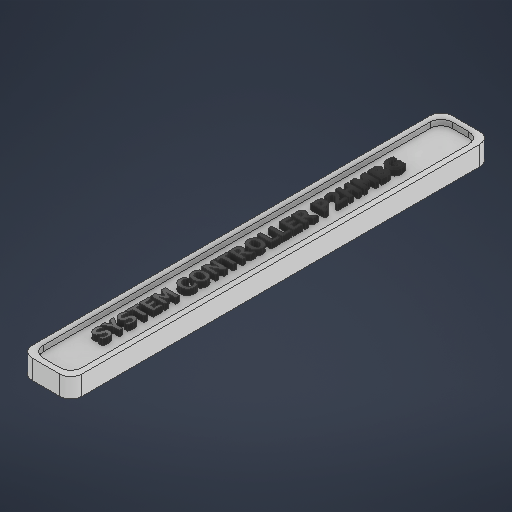
# Autodesk Inventor part: ELEMENT P2HMBG
Saved by Autodesk Inventor 2026.3 (Build 303398000, 398)
## iProperties
Created: 2026-06-09
Part Number: ELEMENT P2HMBG
Material: Generic
Document SubType Name: Modeling
Designer: ilyas
Density: 1 g/cm^3
Appearance: Default
Author: ilyas
Autodesk Inventor part; units mm, degrees
ref_plane "YZ Plane" through (0, 0, 0) normal (1, 0, 0) x (0, 1, 0)
ref_plane "XZ Plane" through (0, 0, 0) normal (0, 1, 0) x (-1, 0, 0)
ref_plane "XY Plane" through (0, 0, 0) normal (0, 0, 1) x (1, 0, 0)
sketch "Sketch1" plane through (0, 0, 0) normal (0, 1, 0) x (-1, 0, 0)
  line L0 (-4.5, 38) -> (4.5, 38)
  line L1 (4.5, 38) -> (4.5, -38)
  line L2 (4.5, -38) -> (-4.5, -38)
  line L3 (-4.5, -38) -> (-4.5, 38)
  line L4 (-4.5, 38) -> (4.5, -38) construction
  line L5 (4.5, 38) -> (-4.5, -38) construction
  point P0 (0, 0)
  dimension "d0" = 9
  dimension "d1" = 76
  constraints: 12 end point, 2 midpoint, 2 parallel, 1 horizontal, 1 perpendicular
  measures "d0" distance of L1.end L2.end
  measures "d1" distance of L0.end L1.end
extrude "Extrusion1" add sketch "Sketch1" along normal blind 2.5
sketch "Sketch2" plane through (0, 2.5, 0) normal (0, 1, 0) x (1, 0, 0)
  line L0 (4.5, -38) -> (-4.5, -38)
  line L1 (-4.5, -38) -> (-4.5, 38)
  line L2 (-4.5, 38) -> (4.5, 38)
  line L3 (4.5, 38) -> (4.5, -38)
  line L4 (4.5, -38) -> (-4.5, 38) construction
  line L5 (-4.5, -38) -> (4.5, 38) construction
  line L6 (-3.5, 37) -> (-3.5, -37)
  line L7 (-3.5, -37) -> (3.5, -37)
  line L8 (3.5, -37) -> (3.5, 37)
  line L9 (3.5, 37) -> (-3.5, 37)
  point P0 (0, 0)
  dimension "d4" = 9
  dimension "d5" = 76
  dimension "d6" = 1
  constraints: 20 end point, 4 parallel, 2 midpoint, 2 perpendicular, 1 horizontal, 3 other
  measures "d4" distance of L1.end L2.end
  measures "d5" distance of L0.end L1.end
  measures "d6" distance between parallel lines of L1 L6
emboss "Emboss1" sketch "Sketch2" operation add depth 1 direction (0, -1, 0)
sketch "Sketch3" plane through (0, 2.5, 0) normal (0, 1, 0) x (1, 0, 0)
  line L0 (-7.0021, -29.5186) -> (-7.0021, 27.1388) construction
  line L1 (-7.0021, 27.1388) -> (6.5444, 27.1388) construction
  line L2 (6.5444, 27.1388) -> (6.5444, -29.5186) construction
  line L3 (6.5444, -29.5186) -> (-7.0021, -29.5186) construction
  spline S0 degree 2 poles (1.0865, -27.7879) (1.0865, -28.0801) (0.9732, -28.5206) (0.8909, -28.71) knots 0 0 0 1 2 2 2
  line L4 (0.8909, -28.71) -> (0.2858, -28.71)
  line L5 (0.2858, -28.71) -> (0.2858, -28.6524)
  spline S1 degree 2 poles (0.2858, -28.6524) (0.4484, -28.4609) (0.6233, -28.0019) (0.6233, -27.7858) knots 0 0 0 1 2 2 2
  spline S2 degree 2 poles (0.6233, -27.7858) (0.6233, -27.7302) (0.5986, -27.5511) (0.5739, -27.4976) knots 0 0 0 1 2 2 2
  spline S3 degree 2 poles (0.5739, -27.4976) (0.5451, -27.4318) (0.4401, -27.3391) (0.3557, -27.3391) knots 0 0 0 1 2 2 2
  spline S4 degree 2 poles (0.3557, -27.3391) (0.259, -27.3391) (0.1396, -27.4894) (0.1129, -27.5923) knots 0 0 0 1 2 2 2
  spline S5 degree 2 poles (0.1129, -27.5923) (0.0779, -27.722) (0.0182, -28.0163) (-0.0271, -28.146) knots 0 0 0 1 2 2 2
  spline S6 degree 2 poles (-0.0271, -28.146) (-0.13, -28.4404) (-0.482, -28.6956) (-0.7455, -28.6956) knots 0 0 0 1 2 2 2
  spline S7 degree 2 poles (-0.7455, -28.6956) (-1.1016, -28.6956) (-1.5441, -28.0925) (-1.5441, -27.6397) knots 0 0 0 1 2 2 2
  spline S8 degree 2 poles (-1.5441, -27.6397) (-1.5441, -27.4132) (-1.4515, -26.9645) (-1.3733, -26.7875) knots 0 0 0 1 2 2 2
  line L6 (-1.3733, -26.7875) -> (-0.7928, -26.7875)
  line L7 (-0.7928, -26.7875) -> (-0.7928, -26.8431)
  spline S9 degree 2 poles (-0.7928, -26.8431) (-0.9143, -26.9851) (-1.081, -27.3927) (-1.081, -27.6067) knots 0 0 0 1 2 2 2
  spline S10 degree 2 poles (-1.081, -27.6067) (-1.081, -27.6911) (-1.0563, -27.8228) (-1.0233, -27.8969) knots 0 0 0 1 2 2 2
  spline S11 degree 2 poles (-1.0233, -27.8969) (-0.9966, -27.9566) (-0.8896, -28.0431) (-0.8237, -28.0431) knots 0 0 0 1 2 2 2
  spline S12 degree 2 poles (-0.8237, -28.0431) (-0.7249, -28.0431) (-0.6117, -27.9052) (-0.5664, -27.7076) knots 0 0 0 1 2 2 2
  spline S13 degree 2 poles (-0.5664, -27.7076) (-0.5376, -27.58) (-0.482, -27.3433) (-0.4347, -27.2074) knots 0 0 0 1 2 2 2
  spline S14 degree 2 poles (-0.4347, -27.2074) (-0.3379, -26.9439) (-0.0168, -26.6866) (0.2467, -26.6866) knots 0 0 0 1 2 2 2
  spline S15 degree 2 poles (0.2467, -26.6866) (0.6254, -26.6866) (1.0865, -27.2815) (1.0865, -27.7879) knots 0 0 0 1 2 2 2
  line L8 (-1.4988, -24.2475) -> (-0.0189, -25.1244)
  line L9 (-0.0189, -25.1244) -> (1.0412, -25.1244)
  line L10 (1.0412, -25.1244) -> (1.0412, -25.7624)
  line L11 (1.0412, -25.7624) -> (0.012, -25.7624)
  line L12 (0.012, -25.7624) -> (-1.4988, -26.6537)
  line L13 (-1.4988, -26.6537) -> (-1.4988, -25.9271)
  line L14 (-1.4988, -25.9271) -> (-0.5932, -25.431)
  line L15 (-0.5932, -25.431) -> (-1.4988, -24.9515)
  line L16 (-1.4988, -24.9515) -> (-1.4988, -24.2475)
  spline S16 degree 2 poles (1.0865, -23.2327) (1.0865, -23.525) (0.9732, -23.9655) (0.8909, -24.1549) knots 0 0 0 1 2 2 2
  line L17 (0.8909, -24.1549) -> (0.2858, -24.1549)
  line L18 (0.2858, -24.1549) -> (0.2858, -24.0972)
  spline S17 degree 2 poles (0.2858, -24.0972) (0.4484, -23.9058) (0.6233, -23.4468) (0.6233, -23.2307) knots 0 0 0 1 2 2 2
  spline S18 degree 2 poles (0.6233, -23.2307) (0.6233, -23.1751) (0.5986, -22.996) (0.5739, -22.9425) knots 0 0 0 1 2 2 2
  spline S19 degree 2 poles (0.5739, -22.9425) (0.5451, -22.8766) (0.4401, -22.784) (0.3557, -22.784) knots 0 0 0 1 2 2 2
  spline S20 degree 2 poles (0.3557, -22.784) (0.259, -22.784) (0.1396, -22.9343) (0.1129, -23.0372) knots 0 0 0 1 2 2 2
  spline S21 degree 2 poles (0.1129, -23.0372) (0.0779, -23.1669) (0.0182, -23.4612) (-0.0271, -23.5909) knots 0 0 0 1 2 2 2
  spline S22 degree 2 poles (-0.0271, -23.5909) (-0.13, -23.8852) (-0.482, -24.1405) (-0.7455, -24.1405) knots 0 0 0 1 2 2 2
  spline S23 degree 2 poles (-0.7455, -24.1405) (-1.1016, -24.1405) (-1.5441, -23.5374) (-1.5441, -23.0845) knots 0 0 0 1 2 2 2
  spline S24 degree 2 poles (-1.5441, -23.0845) (-1.5441, -22.8581) (-1.4515, -22.4094) (-1.3733, -22.2324) knots 0 0 0 1 2 2 2
  line L19 (-1.3733, -22.2324) -> (-0.7928, -22.2324)
  line L20 (-0.7928, -22.2324) -> (-0.7928, -22.288)
  spline S25 degree 2 poles (-0.7928, -22.288) (-0.9143, -22.43) (-1.081, -22.8375) (-1.081, -23.0516) knots 0 0 0 1 2 2 2
  spline S26 degree 2 poles (-1.081, -23.0516) (-1.081, -23.136) (-1.0563, -23.2677) (-1.0233, -23.3418) knots 0 0 0 1 2 2 2
  spline S27 degree 2 poles (-1.0233, -23.3418) (-0.9966, -23.4015) (-0.8896, -23.488) (-0.8237, -23.488) knots 0 0 0 1 2 2 2
  spline S28 degree 2 poles (-0.8237, -23.488) (-0.7249, -23.488) (-0.6117, -23.3501) (-0.5664, -23.1525) knots 0 0 0 1 2 2 2
  spline S29 degree 2 poles (-0.5664, -23.1525) (-0.5376, -23.0248) (-0.482, -22.7881) (-0.4347, -22.6523) knots 0 0 0 1 2 2 2
  spline S30 degree 2 poles (-0.4347, -22.6523) (-0.3379, -22.3888) (-0.0168, -22.1315) (0.2467, -22.1315) knots 0 0 0 1 2 2 2
  spline S31 degree 2 poles (0.2467, -22.1315) (0.6254, -22.1315) (1.0865, -22.7264) (1.0865, -23.2327) knots 0 0 0 1 2 2 2
  line L21 (1.0412, -21.3164) -> (-1.0151, -21.3164)
  line L22 (-1.0151, -21.3164) -> (-1.0151, -22.0677)
  line L23 (-1.0151, -22.0677) -> (-1.4988, -22.0677)
  line L24 (-1.4988, -22.0677) -> (-1.4988, -19.927)
  line L25 (-1.4988, -19.927) -> (-1.0151, -19.927)
  line L26 (-1.0151, -19.927) -> (-1.0151, -20.6783)
  line L27 (-1.0151, -20.6783) -> (1.0412, -20.6783)
  line L28 (1.0412, -20.6783) -> (1.0412, -21.3164)
  line L29 (1.0412, -19.6656) -> (-1.4988, -19.6656)
  line L30 (-1.4988, -19.6656) -> (-1.4988, -17.949)
  line L31 (-1.4988, -17.949) -> (-1.0151, -17.949)
  line L32 (-1.0151, -17.949) -> (-1.0151, -19.0316)
  line L33 (-1.0151, -19.0316) -> (-0.5685, -19.0316)
  line L34 (-0.5685, -19.0316) -> (-0.5685, -18.0333)
  line L35 (-0.5685, -18.0333) -> (-0.0847, -18.0333)
  line L36 (-0.0847, -18.0333) -> (-0.0847, -19.0316)
  line L37 (-0.0847, -19.0316) -> (0.5575, -19.0316)
  line L38 (0.5575, -19.0316) -> (0.5575, -17.949)
  line L39 (0.5575, -17.949) -> (1.0412, -17.949)
  line L40 (1.0412, -17.949) -> (1.0412, -19.6656)
  line L41 (1.0412, -14.9232) -> (1.0412, -15.5572)
  line L42 (1.0412, -15.5572) -> (-0.6426, -15.5572)
  line L43 (-0.6426, -15.5572) -> (0.4443, -16.0182)
  line L44 (0.4443, -16.0182) -> (0.4443, -16.4546)
  line L45 (0.4443, -16.4546) -> (-0.6426, -16.9157)
  line L46 (-0.6426, -16.9157) -> (1.0412, -16.9157)
  line L47 (1.0412, -16.9157) -> (1.0412, -17.5167)
  line L48 (1.0412, -17.5167) -> (-1.4988, -17.5167)
  line L49 (-1.4988, -17.5167) -> (-1.4988, -16.7819)
  line L50 (-1.4988, -16.7819) -> (-0.2453, -16.2179)
  line L51 (-0.2453, -16.2179) -> (-1.4988, -15.658)
  line L52 (-1.4988, -15.658) -> (-1.4988, -14.9232)
  line L53 (-1.4988, -14.9232) -> (1.0412, -14.9232)
  spline S32 degree 2 poles (1.0906, -12.2782) (1.0906, -12.8504) (0.399, -13.5215) (-0.2268, -13.5215) knots 0 0 0 1 2 2 2
  spline S33 degree 2 poles (-0.2268, -13.5215) (-0.8299, -13.5215) (-1.5482, -12.8484) (-1.5482, -12.2762) knots 0 0 0 1 2 2 2
  spline S34 degree 2 poles (-1.5482, -12.2762) (-1.5482, -12.1259) (-1.5132, -11.883) (-1.4844, -11.7719) knots 0 0 0 1 2 2 2
  spline S35 degree 2 poles (-1.4844, -11.7719) (-1.4577, -11.6854) (-1.3692, -11.4816) (-1.3362, -11.4178) knots 0 0 0 1 2 2 2
  line L54 (-1.3362, -11.4178) -> (-0.7311, -11.4178)
  line L55 (-0.7311, -11.4178) -> (-0.7311, -11.4816)
  spline S36 degree 2 poles (-0.7311, -11.4816) (-0.7722, -11.529) (-0.8875, -11.6689) (-0.941, -11.7575) knots 0 0 0 1 2 2 2
  spline S37 degree 2 poles (-0.941, -11.7575) (-0.9966, -11.846) (-1.0727, -12.058) (-1.0727, -12.1753) knots 0 0 0 1 2 2 2
  spline S38 degree 2 poles (-1.0727, -12.1753) (-1.0727, -12.3132) (-0.9863, -12.5417) (-0.8772, -12.6467) knots 0 0 0 1 2 2 2
  spline S39 degree 2 poles (-0.8772, -12.6467) (-0.7805, -12.7413) (-0.4491, -12.8628) (-0.2247, -12.8628) knots 0 0 0 1 2 2 2
  spline S40 degree 2 poles (-0.2247, -12.8628) (0.012, -12.8628) (0.3352, -12.7372) (0.434, -12.6343) knots 0 0 0 1 2 2 2
  spline S41 degree 2 poles (0.434, -12.6343) (0.5307, -12.5355) (0.6151, -12.2926) (0.6151, -12.1712) knots 0 0 0 1 2 2 2
  spline S42 degree 2 poles (0.6151, -12.1712) (0.6151, -12.0456) (0.5307, -11.8171) (0.4792, -11.7389) knots 0 0 0 1 2 2 2
  spline S43 degree 2 poles (0.4792, -11.7389) (0.4278, -11.6525) (0.3187, -11.5228) (0.2755, -11.4755) knots 0 0 0 1 2 2 2
  line L56 (0.2755, -11.4755) -> (0.2755, -11.4178)
  line L57 (0.2755, -11.4178) -> (0.8724, -11.4178)
  spline S44 degree 2 poles (0.8724, -11.4178) (0.9053, -11.4878) (0.9877, -11.671) (1.0165, -11.7698) knots 0 0 0 1 2 2 2
  spline S45 degree 2 poles (1.0165, -11.7698) (1.0535, -11.8892) (1.0906, -12.0971) (1.0906, -12.2782) knots 0 0 0 1 2 2 2
  spline S46 degree 2 poles (-0.2288, -8.7296) (0.3887, -8.7296) (1.0947, -9.3883) (1.0947, -9.9605) knots 0 0 0 1 2 2 2
  spline S47 degree 2 poles (1.0947, -9.9605) (1.0947, -10.5348) (0.3804, -11.1893) (-0.2288, -11.1893) knots 0 0 0 1 2 2 2
  spline S48 degree 2 poles (-0.2288, -11.1893) (-0.8402, -11.1893) (-1.5523, -10.5348) (-1.5523, -9.9605) knots 0 0 0 1 2 2 2
  spline S49 degree 2 poles (-1.5523, -9.9605) (-1.5523, -9.3883) (-0.8443, -8.7296) (-0.2288, -8.7296) knots 0 0 0 1 2 2 2
  spline S50 degree 2 poles (-0.2288, -9.3883) (-0.4573, -9.3883) (-0.7763, -9.4809) (-0.8772, -9.5612) knots 0 0 0 1 2 2 2
  spline S51 degree 2 poles (-0.8772, -9.5612) (-0.9822, -9.6415) (-1.0727, -9.8473) (-1.0727, -9.9585) knots 0 0 0 1 2 2 2
  spline S52 degree 2 poles (-1.0727, -9.9585) (-1.0727, -10.0758) (-0.9884, -10.2672) (-0.8813, -10.3557) knots 0 0 0 1 2 2 2
  spline S53 degree 2 poles (-0.8813, -10.3557) (-0.7825, -10.4339) (-0.4552, -10.5307) (-0.2288, -10.5307) knots 0 0 0 1 2 2 2
  spline S54 degree 2 poles (-0.2288, -10.5307) (0.0058, -10.5307) (0.3146, -10.438) (0.4196, -10.3578) knots 0 0 0 1 2 2 2
  spline S55 degree 2 poles (0.4196, -10.3578) (0.5245, -10.2775) (0.6151, -10.0696) (0.6151, -9.9585) knots 0 0 0 1 2 2 2
  spline S56 degree 2 poles (0.6151, -9.9585) (0.6151, -9.8452) (0.5184, -9.6353) (0.4154, -9.5591) knots 0 0 0 1 2 2 2
  spline S57 degree 2 poles (0.4154, -9.5591) (0.3043, -9.4768) (0.0099, -9.3883) (-0.2288, -9.3883) knots 0 0 0 1 2 2 2
  line L58 (1.0412, -6.1752) -> (1.0412, -6.7886)
  line L59 (1.0412, -6.7886) -> (-0.729, -7.7684)
  line L60 (-0.729, -7.7684) -> (1.0412, -7.7684)
  line L61 (1.0412, -7.7684) -> (1.0412, -8.3509)
  line L62 (1.0412, -8.3509) -> (-1.4988, -8.3509)
  line L63 (-1.4988, -8.3509) -> (-1.4988, -7.5687)
  line L64 (-1.4988, -7.5687) -> (-0.0436, -6.7577)
  line L65 (-0.0436, -6.7577) -> (-1.4988, -6.7577)
  line L66 (-1.4988, -6.7577) -> (-1.4988, -6.1752)
  line L67 (-1.4988, -6.1752) -> (1.0412, -6.1752)
  line L68 (1.0412, -5.1707) -> (-1.0151, -5.1707)
  line L69 (-1.0151, -5.1707) -> (-1.0151, -5.922)
  line L70 (-1.0151, -5.922) -> (-1.4988, -5.922)
  line L71 (-1.4988, -5.922) -> (-1.4988, -3.7814)
  line L72 (-1.4988, -3.7814) -> (-1.0151, -3.7814)
  line L73 (-1.0151, -3.7814) -> (-1.0151, -4.5327)
  line L74 (-1.0151, -4.5327) -> (1.0412, -4.5327)
  line L75 (1.0412, -4.5327) -> (1.0412, -5.1707)
  line L76 (1.0412, -1.1734) -> (1.0412, -1.9494)
  line L77 (1.0412, -1.9494) -> (0.1087, -2.6554)
  line L78 (0.1087, -2.6554) -> (0.1087, -2.886)
  line L79 (0.1087, -2.886) -> (1.0412, -2.886)
  line L80 (1.0412, -2.886) -> (1.0412, -3.5199)
  line L81 (1.0412, -3.5199) -> (-1.4988, -3.5199)
  line L82 (-1.4988, -3.5199) -> (-1.4988, -2.499)
  spline S58 degree 2 poles (-1.4988, -2.499) (-1.4988, -2.287) (-1.4453, -1.9741) (-1.363, -1.8403) knots 0 0 0 1 2 2 2
  spline S59 degree 2 poles (-1.363, -1.8403) (-1.2765, -1.7045) (-1.0069, -1.5439) (-0.801, -1.5439) knots 0 0 0 1 2 2 2
  spline S60 degree 2 poles (-0.801, -1.5439) (-0.5108, -1.5439) (-0.1465, -1.8074) (-0.0395, -2.0276) knots 0 0 0 1 2 2 2
  line L83 (-0.0395, -2.0276) -> (1.0412, -1.1734)
  spline S61 degree 2 poles (-0.7208, -2.1985) (-0.8175, -2.1985) (-0.9554, -2.2726) (-0.9925, -2.357) knots 0 0 0 1 2 2 2
  spline S62 degree 2 poles (-0.9925, -2.357) (-1.0172, -2.4167) (-1.0316, -2.5628) (-1.0316, -2.6719) knots 0 0 0 1 2 2 2
  line L84 (-1.0316, -2.6719) -> (-1.0316, -2.886)
  line L85 (-1.0316, -2.886) -> (-0.3482, -2.886)
  line L86 (-0.3482, -2.886) -> (-0.3482, -2.7028)
  spline S63 degree 2 poles (-0.3482, -2.7028) (-0.3482, -2.571) (-0.3811, -2.3837) (-0.4326, -2.3199) knots 0 0 0 1 2 2 2
  spline S64 degree 2 poles (-0.4326, -2.3199) (-0.482, -2.2582) (-0.6137, -2.1985) (-0.7208, -2.1985) knots 0 0 0 1 2 2 2
  spline S65 degree 2 poles (-0.2288, 1.3275) (0.3887, 1.3275) (1.0947, 0.6688) (1.0947, 0.0966) knots 0 0 0 1 2 2 2
  spline S66 degree 2 poles (1.0947, 0.0966) (1.0947, -0.4777) (0.3804, -1.1323) (-0.2288, -1.1323) knots 0 0 0 1 2 2 2
  spline S67 degree 2 poles (-0.2288, -1.1323) (-0.8402, -1.1323) (-1.5523, -0.4777) (-1.5523, 0.0966) knots 0 0 0 1 2 2 2
  spline S68 degree 2 poles (-1.5523, 0.0966) (-1.5523, 0.6688) (-0.8443, 1.3275) (-0.2288, 1.3275) knots 0 0 0 1 2 2 2
  spline S69 degree 2 poles (-0.2288, 0.6688) (-0.4573, 0.6688) (-0.7763, 0.5762) (-0.8772, 0.4959) knots 0 0 0 1 2 2 2
  spline S70 degree 2 poles (-0.8772, 0.4959) (-0.9822, 0.4156) (-1.0727, 0.2098) (-1.0727, 0.0986) knots 0 0 0 1 2 2 2
  spline S71 degree 2 poles (-1.0727, 0.0986) (-1.0727, -0.0187) (-0.9884, -0.2101) (-0.8813, -0.2986) knots 0 0 0 1 2 2 2
  spline S72 degree 2 poles (-0.8813, -0.2986) (-0.7825, -0.3769) (-0.4552, -0.4736) (-0.2288, -0.4736) knots 0 0 0 1 2 2 2
  spline S73 degree 2 poles (-0.2288, -0.4736) (0.0058, -0.4736) (0.3146, -0.381) (0.4196, -0.3007) knots 0 0 0 1 2 2 2
  spline S74 degree 2 poles (0.4196, -0.3007) (0.5245, -0.2204) (0.6151, -0.0125) (0.6151, 0.0986) knots 0 0 0 1 2 2 2
  spline S75 degree 2 poles (0.6151, 0.0986) (0.6151, 0.2118) (0.5184, 0.4218) (0.4154, 0.4979) knots 0 0 0 1 2 2 2
  spline S76 degree 2 poles (0.4154, 0.4979) (0.3043, 0.5803) (0.0099, 0.6688) (-0.2288, 0.6688) knots 0 0 0 1 2 2 2
  line L87 (1.0412, 3.4002) -> (1.0412, 1.7062)
  line L88 (1.0412, 1.7062) -> (-1.4988, 1.7062)
  line L89 (-1.4988, 1.7062) -> (-1.4988, 2.3443)
  line L90 (-1.4988, 2.3443) -> (0.5575, 2.3443)
  line L91 (0.5575, 2.3443) -> (0.5575, 3.4002)
  line L92 (0.5575, 3.4002) -> (1.0412, 3.4002)
  line L93 (1.0412, 5.3989) -> (1.0412, 3.7049)
  line L94 (1.0412, 3.7049) -> (-1.4988, 3.7049)
  line L95 (-1.4988, 3.7049) -> (-1.4988, 4.3429)
  line L96 (-1.4988, 4.3429) -> (0.5575, 4.3429)
  line L97 (0.5575, 4.3429) -> (0.5575, 5.3989)
  line L98 (0.5575, 5.3989) -> (1.0412, 5.3989)
  line L99 (1.0412, 5.7035) -> (-1.4988, 5.7035)
  line L100 (-1.4988, 5.7035) -> (-1.4988, 7.4202)
  line L101 (-1.4988, 7.4202) -> (-1.0151, 7.4202)
  line L102 (-1.0151, 7.4202) -> (-1.0151, 6.3375)
  line L103 (-1.0151, 6.3375) -> (-0.5685, 6.3375)
  line L104 (-0.5685, 6.3375) -> (-0.5685, 7.3358)
  line L105 (-0.5685, 7.3358) -> (-0.0847, 7.3358)
  line L106 (-0.0847, 7.3358) -> (-0.0847, 6.3375)
  line L107 (-0.0847, 6.3375) -> (0.5575, 6.3375)
  line L108 (0.5575, 6.3375) -> (0.5575, 7.4202)
  line L109 (0.5575, 7.4202) -> (1.0412, 7.4202)
  line L110 (1.0412, 7.4202) -> (1.0412, 5.7035)
  line L111 (1.0412, 10.1989) -> (1.0412, 9.4229)
  line L112 (1.0412, 9.4229) -> (0.1087, 8.7169)
  line L113 (0.1087, 8.7169) -> (0.1087, 8.4864)
  line L114 (0.1087, 8.4864) -> (1.0412, 8.4864)
  line L115 (1.0412, 8.4864) -> (1.0412, 7.8524)
  line L116 (1.0412, 7.8524) -> (-1.4988, 7.8524)
  line L117 (-1.4988, 7.8524) -> (-1.4988, 8.8734)
  spline S77 degree 2 poles (-1.4988, 8.8734) (-1.4988, 9.0854) (-1.4453, 9.3982) (-1.363, 9.532) knots 0 0 0 1 2 2 2
  spline S78 degree 2 poles (-1.363, 9.532) (-1.2765, 9.6679) (-1.0069, 9.8284) (-0.801, 9.8284) knots 0 0 0 1 2 2 2
  spline S79 degree 2 poles (-0.801, 9.8284) (-0.5108, 9.8284) (-0.1465, 9.565) (-0.0395, 9.3447) knots 0 0 0 1 2 2 2
  line L118 (-0.0395, 9.3447) -> (1.0412, 10.1989)
  spline S80 degree 2 poles (-0.7208, 9.1739) (-0.8175, 9.1739) (-0.9554, 9.0998) (-0.9925, 9.0154) knots 0 0 0 1 2 2 2
  spline S81 degree 2 poles (-0.9925, 9.0154) (-1.0172, 8.9557) (-1.0316, 8.8096) (-1.0316, 8.7005) knots 0 0 0 1 2 2 2
  line L119 (-1.0316, 8.7005) -> (-1.0316, 8.4864)
  line L120 (-1.0316, 8.4864) -> (-0.3482, 8.4864)
  line L121 (-0.3482, 8.4864) -> (-0.3482, 8.6696)
  spline S82 degree 2 poles (-0.3482, 8.6696) (-0.3482, 8.8013) (-0.3811, 8.9886) (-0.4326, 9.0524) knots 0 0 0 1 2 2 2
  spline S83 degree 2 poles (-0.4326, 9.0524) (-0.482, 9.1142) (-0.6137, 9.1739) (-0.7208, 9.1739) knots 0 0 0 1 2 2 2
  spline S84 degree 2 poles (-0.6981, 13.3647) (-0.5211, 13.3647) (-0.2, 13.2515) (-0.093, 13.1465) knots 0 0 0 1 2 2 2
  spline S85 degree 2 poles (-0.093, 13.1465) (-0.025, 13.0827) (0.0861, 12.9262) (0.1252, 12.8336) knots 0 0 0 1 2 2 2
  spline S86 degree 2 poles (0.1252, 12.8336) (0.1643, 12.7389) (0.2096, 12.5187) (0.2096, 12.3828) knots 0 0 0 1 2 2 2
  line L122 (0.2096, 12.3828) -> (0.2096, 12.0494)
  line L123 (0.2096, 12.0494) -> (1.0412, 12.0494)
  line L124 (1.0412, 12.0494) -> (1.0412, 11.4113)
  line L125 (1.0412, 11.4113) -> (-1.4988, 11.4113)
  line L126 (-1.4988, 11.4113) -> (-1.4988, 12.3973)
  spline S87 degree 2 poles (-1.4988, 12.3973) (-1.4988, 12.6154) (-1.4186, 12.9345) (-1.3321, 13.0642) knots 0 0 0 1 2 2 2
  spline S88 degree 2 poles (-1.3321, 13.0642) (-1.2354, 13.2082) (-0.9184, 13.3647) (-0.6981, 13.3647) knots 0 0 0 1 2 2 2
  spline S89 degree 2 poles (-0.6817, 12.7101) (-0.7908, 12.7101) (-0.9451, 12.6072) (-0.9739, 12.5372) knots 0 0 0 1 2 2 2
  spline S90 degree 2 poles (-0.9739, 12.5372) (-1.0131, 12.4467) (-1.0254, 12.282) (-1.0254, 12.14) knots 0 0 0 1 2 2 2
  line L127 (-1.0254, 12.14) -> (-1.0254, 12.0494)
  line L128 (-1.0254, 12.0494) -> (-0.2638, 12.0494)
  line L129 (-0.2638, 12.0494) -> (-0.2638, 12.0947)
  spline S91 degree 2 poles (-0.2638, 12.0947) (-0.2638, 12.1832) (-0.2679, 12.3437) (-0.2782, 12.4034) knots 0 0 0 1 2 2 2
  spline S92 degree 2 poles (-0.2782, 12.4034) (-0.2865, 12.4549) (-0.3359, 12.5681) (-0.3667, 12.599) knots 0 0 0 1 2 2 2
  spline S93 degree 2 poles (-0.3667, 12.599) (-0.4285, 12.6648) (-0.5664, 12.7101) (-0.6817, 12.7101) knots 0 0 0 1 2 2 2
  line L130 (1.0412, 15.5671) -> (1.0412, 13.7002)
  line L131 (1.0412, 13.7002) -> (0.6274, 13.7002)
  spline S94 degree 2 poles (0.6274, 13.7002) (0.4381, 13.9369) (0.1046, 14.3156) (-0.0456, 14.4577) knots 0 0 0 1 2 2 2
  spline S95 degree 2 poles (-0.0456, 14.4577) (-0.2412, 14.645) (-0.5396, 14.8117) (-0.6961, 14.8117) knots 0 0 0 1 2 2 2
  spline S96 degree 2 poles (-0.6961, 14.8117) (-0.8731, 14.8117) (-1.0625, 14.5997) (-1.0625, 14.4103) knots 0 0 0 1 2 2 2
  spline S97 degree 2 poles (-1.0625, 14.4103) (-1.0625, 14.3136) (-1.0151, 14.1407) (-0.9781, 14.0522) knots 0 0 0 1 2 2 2
  spline S98 degree 2 poles (-0.9781, 14.0522) (-0.939, 13.9657) (-0.8566, 13.8422) (-0.836, 13.8113) knots 0 0 0 1 2 2 2
  line L132 (-0.836, 13.8113) -> (-0.836, 13.7619)
  line L133 (-0.836, 13.7619) -> (-1.3897, 13.7619)
  spline S99 degree 2 poles (-1.3897, 13.7619) (-1.4412, 13.869) (-1.5482, 14.3259) (-1.5482, 14.5379) knots 0 0 0 1 2 2 2
  spline S100 degree 2 poles (-1.5482, 14.5379) (-1.5482, 14.9908) (-1.1448, 15.456) (-0.7805, 15.456) knots 0 0 0 1 2 2 2
  spline S101 degree 2 poles (-0.7805, 15.456) (-0.5561, 15.456) (-0.1239, 15.2439) (0.1232, 14.999) knots 0 0 0 1 2 2 2
  spline S102 degree 2 poles (0.1232, 14.999) (0.2755, 14.8446) (0.5122, 14.5544) (0.5616, 14.4906) knots 0 0 0 1 2 2 2
  line L134 (0.5616, 14.4906) -> (0.5616, 15.5671)
  line L135 (0.5616, 15.5671) -> (1.0412, 15.5671)
  line L136 (1.0412, 18.0742) -> (1.0412, 17.4361)
  line L137 (1.0412, 17.4361) -> (-0.0847, 17.4361)
  line L138 (-0.0847, 17.4361) -> (-0.0847, 16.5695)
  line L139 (-0.0847, 16.5695) -> (1.0412, 16.5695)
  line L140 (1.0412, 16.5695) -> (1.0412, 15.9314)
  line L141 (1.0412, 15.9314) -> (-1.4988, 15.9314)
  line L142 (-1.4988, 15.9314) -> (-1.4988, 16.5695)
  line L143 (-1.4988, 16.5695) -> (-0.5685, 16.5695)
  line L144 (-0.5685, 16.5695) -> (-0.5685, 17.4361)
  line L145 (-0.5685, 17.4361) -> (-1.4988, 17.4361)
  line L146 (-1.4988, 17.4361) -> (-1.4988, 18.0742)
  line L147 (-1.4988, 18.0742) -> (1.0412, 18.0742)
  line L148 (1.0412, 21.1946) -> (1.0412, 20.5607)
  line L149 (1.0412, 20.5607) -> (-0.6426, 20.5607)
  line L150 (-0.6426, 20.5607) -> (0.4443, 20.0996)
  line L151 (0.4443, 20.0996) -> (0.4443, 19.6632)
  line L152 (0.4443, 19.6632) -> (-0.6426, 19.2021)
  line L153 (-0.6426, 19.2021) -> (1.0412, 19.2021)
  line L154 (1.0412, 19.2021) -> (1.0412, 18.6011)
  line L155 (1.0412, 18.6011) -> (-1.4988, 18.6011)
  line L156 (-1.4988, 18.6011) -> (-1.4988, 19.3359)
  line L157 (-1.4988, 19.3359) -> (-0.2453, 19.8999)
  line L158 (-0.2453, 19.8999) -> (-1.4988, 20.4598)
  line L159 (-1.4988, 20.4598) -> (-1.4988, 21.1946)
  line L160 (-1.4988, 21.1946) -> (1.0412, 21.1946)
  spline S103 degree 2 poles (0.2631, 23.7511) (0.4525, 23.7511) (0.7386, 23.607) (0.8333, 23.4876) knots 0 0 0 1 2 2 2
  spline S104 degree 2 poles (0.8333, 23.4876) (0.9465, 23.3435) (1.0412, 23.0019) (1.0412, 22.7363) knots 0 0 0 1 2 2 2
  line L161 (1.0412, 22.7363) -> (1.0412, 21.7216)
  line L162 (1.0412, 21.7216) -> (-1.4988, 21.7216)
  line L163 (-1.4988, 21.7216) -> (-1.4988, 22.6169)
  spline S105 degree 2 poles (-1.4988, 22.6169) (-1.4988, 22.8969) (-1.4556, 23.185) (-1.3877, 23.3106) knots 0 0 0 1 2 2 2
  spline S106 degree 2 poles (-1.3877, 23.3106) (-1.3156, 23.4485) (-1.0686, 23.5823) (-0.9081, 23.5823) knots 0 0 0 1 2 2 2
  spline S107 degree 2 poles (-0.9081, 23.5823) (-0.7228, 23.5823) (-0.4326, 23.3971) (-0.3647, 23.2324) knots 0 0 0 1 2 2 2
  line L164 (-0.3647, 23.2324) -> (-0.3523, 23.2324)
  spline S108 degree 2 poles (-0.3523, 23.2324) (-0.3029, 23.4691) (0.0038, 23.7511) (0.2631, 23.7511) knots 0 0 0 1 2 2 2
  spline S109 degree 2 poles (0.2528, 23.0924) (0.1334, 23.0924) (-0.0003, 22.9977) (-0.0353, 22.9031) knots 0 0 0 1 2 2 2
  spline S110 degree 2 poles (-0.0353, 22.9031) (-0.058, 22.8454) (-0.0621, 22.6416) (-0.0621, 22.4729) knots 0 0 0 1 2 2 2
  line L165 (-0.0621, 22.4729) -> (-0.0621, 22.3555)
  line L166 (-0.0621, 22.3555) -> (0.578, 22.3555)
  line L167 (0.578, 22.3555) -> (0.578, 22.3905)
  spline S111 degree 2 poles (0.578, 22.3905) (0.578, 22.6375) (0.5719, 22.8269) (0.5286, 22.9257) knots 0 0 0 1 2 2 2
  spline S112 degree 2 poles (0.5286, 22.9257) (0.4895, 23.0121) (0.3455, 23.0924) (0.2528, 23.0924) knots 0 0 0 1 2 2 2
  spline S113 degree 2 poles (-0.7825, 22.9339) (-0.8443, 22.9339) (-0.9739, 22.8701) (-1.0028, 22.8043) knots 0 0 0 1 2 2 2
  spline S114 degree 2 poles (-1.0028, 22.8043) (-1.0316, 22.7425) (-1.0357, 22.5696) (-1.0357, 22.3988) knots 0 0 0 1 2 2 2
  line L168 (-1.0357, 22.3988) -> (-1.0357, 22.3555)
  line L169 (-1.0357, 22.3555) -> (-0.4964, 22.3555)
  line L170 (-0.4964, 22.3555) -> (-0.4964, 22.4358)
  spline S115 degree 2 poles (-0.4964, 22.4358) (-0.4964, 22.5984) (-0.5026, 22.7302) (-0.5355, 22.8001) knots 0 0 0 1 2 2 2
  spline S116 degree 2 poles (-0.5355, 22.8001) (-0.5726, 22.8763) (-0.6981, 22.9339) (-0.7825, 22.9339) knots 0 0 0 1 2 2 2
  spline S117 degree 2 poles (0.8971, 26.2376) (0.965, 26.0708) (1.0947, 25.5377) (1.0947, 25.2784) knots 0 0 0 1 2 2 2
  spline S118 degree 2 poles (1.0947, 25.2784) (1.0947, 24.6794) (0.4031, 23.9693) (-0.2309, 23.9693) knots 0 0 0 1 2 2 2
  spline S119 degree 2 poles (-0.2309, 23.9693) (-0.8278, 23.9693) (-1.5482, 24.6794) (-1.5482, 25.2969) knots 0 0 0 1 2 2 2
  spline S120 degree 2 poles (-1.5482, 25.2969) (-1.5482, 25.616) (-1.4268, 26.0153) (-1.3239, 26.2273) knots 0 0 0 1 2 2 2
  line L171 (-1.3239, 26.2273) -> (-0.7269, 26.2273)
  line L172 (-0.7269, 26.2273) -> (-0.7269, 26.1696)
  spline S121 degree 2 poles (-0.7269, 26.1696) (-0.7619, 26.1244) (-0.8957, 25.9515) (-0.941, 25.8691) knots 0 0 0 1 2 2 2
  spline S122 degree 2 poles (-0.941, 25.8691) (-0.9966, 25.7744) (-1.0748, 25.5233) (-1.0748, 25.3834) knots 0 0 0 1 2 2 2
  spline S123 degree 2 poles (-1.0748, 25.3834) (-1.0748, 25.2208) (-0.9719, 24.9511) (-0.8669, 24.8461) knots 0 0 0 1 2 2 2
  spline S124 degree 2 poles (-0.8669, 24.8461) (-0.764, 24.7453) (-0.4491, 24.6279) (-0.2412, 24.6279) knots 0 0 0 1 2 2 2
  spline S125 degree 2 poles (-0.2412, 24.6279) (0.2034, 24.6279) (0.6274, 25.0746) (0.6274, 25.4595) knots 0 0 0 1 2 2 2
  spline S126 degree 2 poles (0.6274, 25.4595) (0.6274, 25.4945) (0.6233, 25.5851) (0.6213, 25.6201) knots 0 0 0 1 2 2 2
  line L173 (0.6213, 25.6201) -> (0.1211, 25.6201)
  line L174 (0.1211, 25.6201) -> (0.1211, 25.1281)
  line L175 (0.1211, 25.1281) -> (-0.3544, 25.1281)
  line L176 (-0.3544, 25.1281) -> (-0.3544, 26.2376)
  line L177 (-0.3544, 26.2376) -> (0.8971, 26.2376)
  point P0 (0, 0)
  constraints: 2 other
emboss "Emboss2" sketch "Sketch3" operation add depth 1 direction (0, -1, 0)
fillet "Fillet1" radius 2 8 edges at (4.5, 1.75, 38) (-4.5, 1.75, 38) (-4.5, 1.75, -38) (4.5, 1.75, -38) (-3.5, 3, 37) (3.5, 3, 37) (3.5, 3, -37) (-3.5, 3, -37)
body "Solid1"
